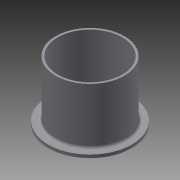
# Autodesk Inventor part: Bearing-Axle Sleeve
Saved by Autodesk Inventor 2014 (Build 180170000, 170)
## iProperties
Created: 2015-02-07
Part Number: Bearing-Axle Sleeve
Material: Generic
Document SubType Name: Modeling
Designer: Spooner
Density: 1 g/cm^3
Appearance: Default
Author: Spooner
Autodesk Inventor part; units mm, degrees
ref_plane "YZ Plane" through (0, 0, 0) normal (1, 0, 0) x (0, 1, 0)
ref_plane "XZ Plane" through (0, 0, 0) normal (0, 1, 0) x (-1, 0, 0)
ref_plane "XY Plane" through (0, 0, 0) normal (0, 0, 1) x (1, 0, 0)
sketch "Sketch1" plane through (0, 0, 0) normal (0, 0, 1) x (1, 0, 0)
  line L0 (-7.874, 0) -> (-7.874, 76.2)
  line L1 (-8.5725, 42.412) -> (8.5725, 42.412) projected
  line L2 (-8.5725, 28.442) -> (-8.5725, 42.412)
  line L3 (-8.5725, 28.442) -> (-10.414, 28.442)
  line L4 (-10.414, 28.442) -> (-10.414, 27.68)
  line L5 (-10.414, 27.68) -> (-7.874, 27.68)
  line L6 (-7.874, 27.68) -> (-7.874, 42.412)
  line L7 (-7.874, 42.412) -> (-8.5725, 42.412)
  line L8 (0, -15.24) -> (0, 91.44) projected
  line L9 (-8.0645, 42.412) -> (-8.0645, 27.68)
  point P0 (0, 0)
  dimension "d0" = 2.54
  dimension "d1" = 0.762
  dimension "d4" = 0.508
  dimension "d5" = 8.0645
  dimension "d6" = 7.874
  constraints: 16 end point, 5 point on line, 3 perpendicular, 2 vertical, 1 collinear, 1 parallel, 3 other
  measures "d0" distance of L4.end L5.end
  measures "d1" distance of L3.end L4.end
  measures "d4" distance between parallel lines of L9 L2
  measures "d5" distance between parallel lines of L8 L9
  measures "d6" distance between parallel lines of L8 L0
revolve "Revolution1" add sketch "Sketch1" angle 360 about axis through (0, -10, 0) along (0, 1, 0) contours L5 L4 L3 L2 L1 L9
fillet "Fillet1" radius 0.635 1 edges at (8.5725, 28.442, 0)
body "Solid1"
